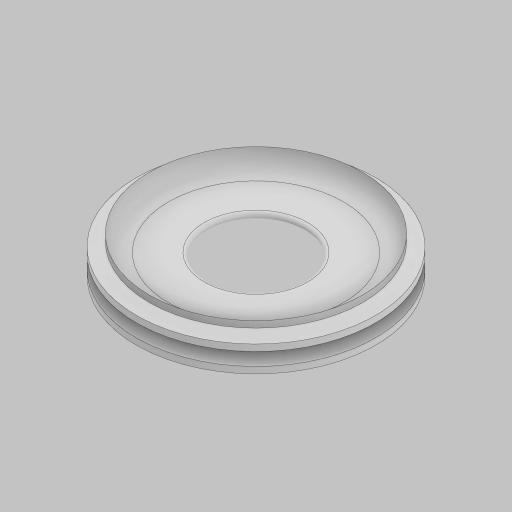
# Autodesk Inventor part: Sealingring
Saved by Autodesk Inventor 2023.2 (Build 272271000, 271)
## iProperties
Created: 2023-02-14
Part Number: Sealingring
Material: Generic
Document SubType Name: Modeling
Designer: splath
Density: 1 g/cm^3
Appearance: Default
Author: splath
Autodesk Inventor part; units mm, degrees
ref_plane "YZ Plane" through (0, 0, 0) normal (1, 0, 0) x (0, 1, 0)
ref_plane "XZ Plane" through (0, 0, 0) normal (0, 1, 0) x (-1, 0, 0)
ref_plane "XY Plane" through (0, 0, 0) normal (0, 0, 1) x (1, 0, 0)
sketch "Sketch1" plane through (0, 0, 0) normal (0, 0, 1) x (1, 0, 0)
  line L0 (-8, -0.5) -> (-13.542, -0.5)
  arc A0 (-8, -0.5) -> (-8, 0.5) centre (-8, 0) ccw
  line L1 (-8, 0.5) -> (-13.542, 0.5)
  arc A1 (-16.5, 3) -> (-13.542, 0.5) centre (-13.542, 3.5) ccw
  line L2 (-16.5, 3) -> (-16.5, 2)
  line L3 (-16.5, 2) -> (-18.5, 1.2721)
  line L4 (-18.5, 1.2721) -> (-18.5, 0.2721)
  line L5 (-18.5, 0.2721) -> (-16.5, 1)
  arc A2 (-13.542, -0.5) -> (-16.5, -3) centre (-13.542, -3.5) ccw
  line L6 (-22.2, 0) -> (3.7, 0) construction
  line L7 (0, -4.9) -> (0, 4.9) construction
  line L8 (-16.5, 1) -> (-16.5, -1)
  line L9 (-16.5, -1) -> (-18.5, -1.7279)
  line L10 (-18.5, -1.7279) -> (-18.5, -2.7279)
  line L11 (-18.5, -2.7279) -> (-16.5, -2)
  line L12 (-16.5, -2) -> (-16.5, -3)
  point P0 (0, 0)
  point P1 (-7.5, 0)
  dimension "d3" = 15
  dimension "d4" = 33
  dimension "d5" = 2
  dimension "d7" = 1
  dimension "d8" = 6
  dimension "d9" = 3
  dimension "d10" = 1
  dimension "d12" = 2
  dimension "d13" = 5.542
  dimension "d15" = 0.7279
  dimension "d16" = 70
  constraints: 22 end point, 7 point on circle, 5 parallel, 4 tangent, 3 centre point, 3 equal length, 3 point on line, 2 horizontal, 2 vertical, 1 collinear, 1 equal radius, 1 perpendicular
  measures "d3" diameter of point (-7.5, 0) L7
  measures "d4" diameter of L2 L7
  measures "d5" distance between parallel lines of L2 L4
  measures "d7" distance between parallel lines of L1 L0
  measures "d8" distance of L12.end L2.start
  measures "d9" radius of A2
  measures "d10" distance of L3.end L4.end
  measures "d12" distance of L5.end L8.end
  measures "d13" distance of L1.start L1.end
  measures "d15" vertical distance of L10.end L11.end
  measures "d16" angle of L11 L12
revolve "Revolution1" add sketch "Sketch1" angle 360 about axis through (0, -10, 0) along (0, 1, 0)
body "Solid1"
